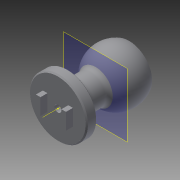
# Autodesk Inventor part: vertebro_back
Saved by Autodesk Inventor 2015 (Build 190159000, 159)
## iProperties
Created: 2014-11-07
Part Number: vertebro_back
Material: Generic
Document SubType Name: Modeling
Designer: Ryan
Density: 1 g/cm^3
Appearance: Default
Author: Ryan
Autodesk Inventor part; units mm, degrees
ref_plane "YZ Plane" through (0, 0, 0) normal (1, 0, 0) x (0, 1, 0)
ref_plane "XZ Plane" through (0, 0, 0) normal (0, 1, 0) x (-1, 0, 0)
ref_plane "XY Plane" through (0, 0, 0) normal (0, 0, 1) x (1, 0, 0)
sketch "Sketch1" plane through (0, 0, 0) normal (1, 0, 0) x (0, 1, 0)
  point P0 (0, 0)
sketch "Sketch2" plane through (0, 0, 0) normal (1, 0, 0) x (0, 1, 0)
  arc A0 (7.8808, -29.55) -> (0, -15.9) centre (0, -25) ccw
  arc A1 (9.9593, -30.75) -> (6.5, -15.5132) centre (0, -25) ccw
  line L0 (0, 0) -> (12.5, 0)
  line L1 (12.5, 0) -> (12.5, -4.5)
  line L2 (12.5, -4.5) -> (6.5, -4.5)
  line L3 (6.5, -4.5) -> (6.5, -15.5132)
  line L4 (7.8808, -29.55) -> (9.9593, -30.75)
  line L5 (0, -15.9) -> (0, 0)
  dimension "d0" = 4.5
  dimension "d2" = 18.2
  dimension "d3" = 23
  dimension "d5" = 25
  dimension "d7" = 12.5
  dimension "d8" = 6.5
  dimension "d9" = 60
  constraints: 12 end point, 4 point on circle, 3 perpendicular, 2 centre point, 2 point on line, 1 coincident, 1 horizontal, 1 vertical
  measures "d0" distance of L0.end L1.end
  measures "d2" diameter of A0
  measures "d3" diameter of A1
  measures "d5" distance of L0.start A0.centre
  measures "d7" distance between parallel lines of L5 L1
  measures "d8" distance between parallel lines of L5 L3
  measures "d9" angle of L5 L4
revolve "Revolution1" add sketch "Sketch2" angle 360 about axis through (0, 0, -15.9) along (0, 0, 1)
hole "Hole1" at (0, 0, 0) direction (0, 0, -1) diameter 3 end through all
ref_plane "Work Plane1" through (0, 0, -16.2) normal (0, 0, -1) x (-1, 0, 0)
sketch "Sketch3" plane through (0, 0, -16.2) normal (0, 0, -1) x (-1, 0, 0)
  circle A0 centre (0, 0) radius 2.3668
  constraints: 1 centre point, 1 coincident
hole "Hole2" at (0, 0, -16.2) direction (0, 0, 1) diameter 4.7336 depth 1.5
chamfer "Chamfer1" distance 0.5 angle 45 1 edges at (0, -12.5, 0)
chamfer "Chamfer2" distance 0.5 angle 45 1 edges at (0, -12.5, -4.5)
fillet "Fillet1" radius 5 1 edges at (0, -6.5, -4.5)
fillet "Fillet2" radius 3 1 edges at (0, -6.5, -15.5132)
sketch "Sketch4" plane through (0, 0, 0) normal (0, 0, 1) x (1, 0, 0)
  line L0 (4.5, -3.5) -> (4.5, 3.5)
  line L1 (4.5, 3.5) -> (6.5, 3.5)
  line L2 (6.5, 3.5) -> (6.5, -3.5)
  line L3 (6.5, -3.5) -> (4.5, -3.5)
  line L4 (-4.5, -3.5) -> (-6.5, -3.5)
  line L5 (-6.5, -3.5) -> (-6.5, 3.5)
  line L6 (-6.5, 3.5) -> (-4.5, 3.5)
  line L7 (-4.5, 3.5) -> (-4.5, -3.5)
  line L8 (0, 0) -> (0, -2.6483) construction
  line L9 (4.5, 0) -> (0, 0) construction
  dimension "d36" = 7
  dimension "d37" = 2
  dimension "d38" = 4.5
  constraints: 20 end point, 6 perpendicular, 2 horizontal, 2 midpoint, 2 vertical, 4 other
  measures "d36" distance of L1.end L2.end
  measures "d37" distance of L2.end L0.start
  measures "d38" distance between parallel lines of L0 L8
extrude "Extrusion1" add sketch "Sketch4" along normal blind 3
body "Solid1"
